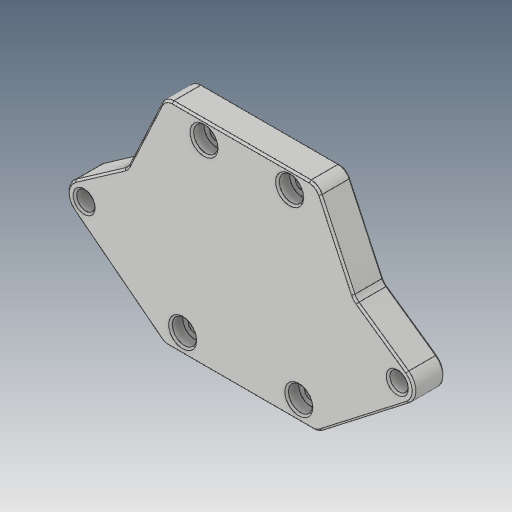
# Autodesk Inventor part: tilt-guide
Saved by Autodesk Inventor 2018 (Build 220112000, 112)
## iProperties
Created: 2019-03-01
Part Number: tilt-guide
Material: Generic
Document SubType Name: Modeling
Designer: Tsche
Density: 1 g/cm^3
Appearance: Default
Author: Tsche
Autodesk Inventor part; units mm, degrees
ref_plane "YZ Plane" through (0, 0, 0) normal (1, 0, 0) x (0, 1, 0)
ref_plane "XZ Plane" through (0, 0, 0) normal (0, 1, 0) x (-1, 0, 0)
ref_plane "XY Plane" through (0, 0, 0) normal (0, 0, 1) x (1, 0, 0)
sketch "Sketch1" plane through (0, 0, 0) normal (0, 0, 1) x (1, 0, 0)
  circle A0 centre (25.625, 0) radius 1.5125
  line L0 (12.5, 21.35) -> (0, 21.35)
  line L1 (0, -20.65) -> (0, 28.35) construction
  line L2 (-39.7989, 0) -> (39.7989, 0) construction
  line L3 (27.3095, -2.1737) -> (12.5, -13.65)
  line L4 (12.5, -13.65) -> (0, -13.65)
  arc A1 (27.3095, -2.1737) -> (27.2023, 2.2527) centre (25.625, 0) ccw
  circle A2 centre (-25.625, 0) radius 1.5125
  line L5 (-12.5, 21.35) -> (0, 21.35)
  line L6 (-27.3095, -2.1737) -> (-12.5, -13.65)
  line L7 (-12.5, -13.65) -> (0, -13.65)
  arc A3 (-27.2023, 2.2527) -> (-27.3095, -2.1737) centre (-25.625, 0) ccw
  line L8 (27.2023, 2.2527) -> (18.625, 8.2586)
  line L9 (18.625, 8.2586) -> (12.5, 21.35)
  line L10 (-27.2023, 2.2527) -> (-18.625, 8.2586)
  line L11 (-18.625, 8.2586) -> (-12.5, 21.35)
  point P0 (0, 0)
  dimension "d0" = 51.25
  dimension "d1" = 3.025
  dimension "d2" = 2.75
  dimension "d84" = 21.35
  dimension "d85" = 13.65
  dimension "d86" = 25
  dimension "d87" = 25
  dimension "d88" = 35
  dimension "d89" = 7
  constraints: 20 end point, 7 symmetric about line, 4 centre point, 4 point on circle, 2 coincident, 2 horizontal, 2 point on line, 2 tangent, 2 other
  measures "d0" distance of A0.centre A3.centre
  measures "d1" diameter of A0
  measures "d2" radius of A1
  measures "d84" distance between parallel lines of L5 L2
  measures "d85" distance between parallel lines of L2 L7
  measures "d86" distance of L3.end L6.end
  measures "d87" distance of L0.start L5.start
  measures "d88" angle of L8 L2
  measures "d89" horizontal distance of L8.end A0.centre
extrude "Extrusion1" add sketch "Sketch1" along normal blind 5
sketch "Sketch4" plane through (0, 0, 5) normal (0, 0, 1) x (1, 0, 0)
  line L0 (-39.725, 0) -> (39.725, 0) construction
  line L1 (0, -20.65) -> (0, 28.35) construction
  point P0 (0, 0)
  point P1 (9.5, -10.5)
  point P2 (8, 18.5)
  point P3 (-6, 18.5)
  point P4 (-9.5, -10.5)
  dimension "d90" = 10.5
  dimension "d91" = 9.5
  dimension "d92" = 18.5
  dimension "d93" = 18.5
  dimension "d94" = 8
  dimension "d95" = 6
  constraints: 1 symmetric about line
  measures "d90" distance from line of L0 point (9.5, -10.5)
  measures "d91" distance from line of L1 point (9.5, -10.5)
  measures "d92" distance from line of L0 point (-6, 18.5)
  measures "d93" distance from line of L0 point (8, 18.5)
  measures "d94" distance from line of L1 point (8, 18.5)
  measures "d95" distance from line of L1 point (-6, 18.5)
hole "Hole2" at (9.5, -10.5, 5) at (8, 18.5, 5) at (-6, 18.5, 5) at (-9.5, -10.5, 5) direction (0, 0, -1) diameter 2.2 end through all counterbore diameter 4 counterbore depth 2
fillet "Fillet5" radius 2 6 edges at (-18.625, 8.2586, 2.5) (18.625, 8.2586, 2.5) (12.5, -13.65, 2.5) (-12.5, -13.65, 2.5) (12.5, 21.35, 2.5) (-12.5, 21.35, 2.5)
chamfer "Chamfer4" distance 0.3 angle 45 44 edges at (0, 21.35, 5) (-12.3012, 21.0375, 5) (-15.7188, 14.4701, 5) (-18.6787, 8.3037, 5) (-23.1326, 5.1023, 5) (-28.3742, 0.0665, 5) (12.3012, 21.0375, 5) (15.7188, 14.4701, 5) (18.6787, 8.3037, 5) (23.1326, 5.1023, 5) (28.3742, 0.0665, 5) (0, 21.35, 0) (12.3012, 21.0375, 0) (15.7188, 14.4701, 0) (18.6787, 8.3037, 0) (23.1326, 5.1023, 0) (28.3742, 0.0665, 0) (-12.3012, 21.0375, 0) (-15.7188, 14.4701, 0) (-18.6787, 8.3037, 0) (-23.1326, 5.1023, 0) (-28.3742, 0.0665, 0) (-20.1752, -7.7023, 5) (-12.4632, -13.5423, 5) (0, -13.65, 5) (12.4632, -13.5423, 5) (20.1752, -7.7023, 5) (-20.1752, -7.7023, 0) (-12.4632, -13.5423, 0) (0, -13.65, 0) (12.4632, -13.5423, 0) (20.1752, -7.7023, 0) (-27.1375, 0, 0) (-9.5, -9.4, 0) (9.5, -9.4, 0) (-6, 19.6, 0) (8, 19.6, 0) (24.1125, 0, 0) (-27.1375, 0, 5) (24.1125, 0, 5) (-9.5, -8.5, 5) (9.5, -8.5, 5) (-6, 20.5, 5) (8, 20.5, 5)
equation "\"d0\" = dist_hinge_points"
equation "\"d1\" = bore_clearance"
equation "\"d104\" = champfer"
equation "\"finger_width\" = 25"
equation "\"finger_thickness\" = 8"
equation "\"finger_part_A_length\" = 42.8625"
equation "\"finger_part_B_length\" = 28.575"
equation "\"finger_link_width\" = 3.5"
equation "\"finger_link_clearence\" = 0.075"
equation "\"tol\" = 0.5 * finger_link_clearence"
equation "\"link_tol\" = 0.254"
equation "\"bore_press\" = 2.925"
equation "\"bore_clearance\" = 3.025"
equation "\"bar_diameter\" = 6.5"
equation "\"bar_thickness\" = 4"
equation "\"bar_width\" = 7"
equation "\"hinge_dist_sym_plane\" = 4"
equation "\"hinge_thickness\" = 3"
equation "\"hinge_act_length_c\" = 7.62"
equation "\"hinge_act_length_bc\" = 16.66875"
equation "\"hinge_act_length_ab\" = 11.049"
equation "\"hinge_act_length_a\" = 21.43125"
equation "\"hinge_guid_length_c\" = 9.525"
equation "\"hinge_guid_length_bc\" = 9.525"
equation "\"hinge_guid_length_ab\" = 17.145"
equation "\"hinge_guid_length_a\" = 17.145"
equation "\"bar_length_bc\" = finger_part_B_length"
equation "\"bar_act_length_ab\" = 40.48125"
equation "\"bar_guid_length_ab\" = 43.275"
equation "\"champfer\" = 0.3"
equation "\"fillet\" = 0.4"
equation "\"hinge_point\" = 15"
equation "\"dist_finger_BC\" = 56.5"
equation "\"gear_diameter\" = 14"
equation "\"dist_hinge_points\" = 51.25"
body "Solid1"
